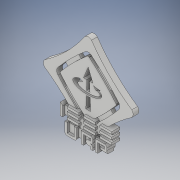
# Autodesk Inventor part: IEEE 3D
Saved by Autodesk Inventor 2018 (Build 220112000, 112)
## iProperties
Created: 2017-04-26
Part Number: IEEE 3D
Material: Generic
Document SubType Name: Modeling
Designer: Docente
Density: 1 g/cm^3
Appearance: Default
Author: Docente
Autodesk Inventor part; units mm, degrees
ref_plane "XY Plane" through (0, 0, 0) normal (0, 0, 1) x (1, 0, 0)
sketch "Sketch1" plane through (0, 0, 0) normal (0, 0, 1) x (1, 0, 0)
  line L0 (0, 0) -> (40, 0) construction
  line L1 (40, 0) -> (40, 40) construction
  line L2 (40, 40) -> (0, 40) construction
  line L3 (0, 40) -> (0, 0) construction
  line L4 (21.4142, 38.5858) -> (38.5858, 21.4142)
  line L5 (21.4142, 1.4142) -> (38.5858, 18.5858)
  line L6 (18.5858, 1.4142) -> (1.4142, 18.5858)
  line L7 (18.5858, 38.5858) -> (1.4142, 21.4142)
  arc A0 (21.4142, 38.5858) -> (18.5858, 38.5858) centre (20, 37.1716) ccw
  arc A1 (38.5858, 18.5858) -> (38.5858, 21.4142) centre (37.1716, 20) ccw
  arc A2 (18.5858, 1.4142) -> (21.4142, 1.4142) centre (20, 2.8284) ccw
  arc A3 (1.4142, 21.4142) -> (1.4142, 18.5858) centre (2.8284, 20) ccw
  line L8 (20, 0) -> (20, 20) construction
  line L9 (20, 20) -> (40, 20) construction
  line L10 (20, 20) -> (76.5685, 76.5685) construction
  line L11 (20, 20) -> (100, 20) construction
  line L12 (20, 20) -> (76.5685, -36.5685) construction
  line L13 (20, 20) -> (100, 20) construction
  line L14 (20, 20) -> (-36.5685, 76.5685) construction
  line L15 (20, 20) -> (100, 20) construction
  line L16 (20, 20) -> (-36.5685, -36.5685) construction
  line L17 (20, 20) -> (100, 20) construction
  line L18 (37.1716, 20) -> (38.5858, 21.4142) construction
  line L19 (37.1716, 20) -> (38.5858, 18.5858) construction
  line L20 (20, 37.1716) -> (21.4142, 38.5858) construction
  line L21 (20, 37.1716) -> (18.5858, 38.5858) construction
  circle A4 centre (76.5685, 76.5685) radius 66.9678
  circle A5 centre (76.5685, -36.5685) radius 66.9678
  circle A6 centre (-36.5685, -36.5685) radius 66.9678
  circle A7 centre (-36.5685, 76.5685) radius 66.9678
  point P0 (20, 40)
  point P1 (20, 0)
  point P2 (0, 20)
  dimension "d0" = 40
  dimension "d1" = 40
  dimension "d7" = 2
  dimension "d8" = 20
  dimension "d13" = 20
  dimension "d14" = 80
  dimension "d15" = 45
  dimension "d16" = 80
  dimension "d17" = 45
  dimension "d18" = 80
  dimension "d19" = 135
  dimension "d20" = 80
  dimension "d21" = 135
  constraints: 44 end point, 8 point on circle, 8 point on line, 8 tangent, 5 horizontal, 4 centre point, 4 coincident, 4 equal length, 4 midpoint, 3 equal radius, 2 parallel, 2 perpendicular, 1 vertical, 12 other
  measures "d0" distance of L2.end L1.end
  measures "d1" distance of L1.end L0.end
  measures "d7" radius of A0
  measures "d8" distance between parallel lines of L3 L8
  measures "d13" distance between parallel lines of L0 L9
  measures "d14" distance of L8.end L10.end
  measures "d15" angle of L11 L10
  measures "d16" distance of L8.end L12.end
  measures "d17" angle of L12 L13
  measures "d18" distance of L8.end L14.end
  measures "d19" angle of L15 L14
  measures "d20" distance of L8.end L16.end
  measures "d21" angle of L16 L17
extrude "Extrusion3" add sketch "Sketch1" along normal blind 2.5 contours A4 A1 A5 A2 A6 A3 A7 A0 | L4 A4 | A7 L7 | L5 A5 | A6 L6
extrude "Extrusion4" cut sketch "Sketch1" along normal blind 3.5 contours A4 A7 A5 L4 | L4 A4 | A7 L7 | L7 A7 A6 A4 | A4 A7 | A5 A4 A6 L5 | L5 A5 | A5 A4 | A6 L6 | L6 A6 A5 A7 | A7 A6 | A6 A5
ref_plane "Work Plane1" through (20, 0, 0) normal (1, 0, 0) x (0, 1, 0)
sketch "Sketch6" plane through (0, 0, 2.5) normal (0, 0, 1) x (1, 0, 0)
  line L0 (18.5858, 38.5858) -> (1.4142, 21.4142) construction
  line L1 (18.5858, 1.4142) -> (1.4142, 18.5858) construction
  line L2 (21.4142, 1.4142) -> (38.5858, 18.5858) construction
  line L3 (21.4142, 38.5858) -> (38.5858, 21.4142) construction
  arc A0 (21.4142, 38.5858) -> (18.5858, 38.5858) centre (20, 37.1716) ccw construction
  arc A1 (1.4142, 21.4142) -> (1.4142, 18.5858) centre (2.8284, 20) ccw construction
  arc A2 (18.5858, 1.4142) -> (21.4142, 1.4142) centre (20, 2.8284) ccw construction
  arc A3 (38.5858, 18.5858) -> (38.5858, 21.4142) centre (37.1716, 20) ccw construction
  line L4 (2.8284, 20) -> (20, 37.1716) construction
  line L5 (20, 37.1716) -> (37.1716, 20) construction
  line L6 (20, 2.8284) -> (37.1716, 20) construction
  line L7 (20, 2.8284) -> (2.8284, 20) construction
  line L8 (18.5858, 32.9289) -> (7.0711, 21.4142) construction
  line L9 (7.0711, 18.5858) -> (18.5858, 7.0711) construction
  line L10 (21.4142, 7.0711) -> (32.9289, 18.5858) construction
  line L11 (32.9289, 21.4142) -> (21.4142, 32.9289) construction
  arc A4 (21.4142, 32.9289) -> (18.8688, 33.1641) centre (20, 31.5147) ccw
  arc A5 (33.1641, 18.8688) -> (33.1641, 21.1312) centre (31.5147, 20) ccw
  arc A6 (18.8688, 6.8359) -> (21.4142, 7.0711) centre (20, 8.4853) ccw
  arc A7 (7.0711, 21.4142) -> (7.0711, 18.5858) centre (8.4853, 20) ccw
  line L12 (20, 31.5147) -> (20, 8.4853) construction
  line L13 (8.4853, 20) -> (31.5147, 20) construction
  line L14 (20, 20) -> (76.5685, 76.5685) construction
  line L15 (20, 20) -> (100, 20) construction
  arc A8 (7.0711, 18.5858) -> (18.8688, 6.8359) centre (76.5685, 76.5685) ccw
  line L16 (20, 20) -> (-36.5685, 76.5685) construction
  arc A9 (21.4142, 7.0711) -> (33.1641, 18.8688) centre (-36.5685, 76.5685) ccw
  line L17 (20, 20) -> (-36.5685, -36.5685) construction
  line L18 (20, 20) -> (76.5685, -36.5685) construction
  arc A10 (18.8688, 33.1641) -> (7.0711, 21.4142) centre (76.5685, -36.5685) ccw
  arc A11 (33.1641, 21.1312) -> (21.4142, 32.9289) centre (-36.5685, -36.5685) ccw
  point P0 (0, 0)
  dimension "d41" = 2
  dimension "d42" = 2
  dimension "d43" = 80
  dimension "d44" = 45
  constraints: 30 end point, 16 point on circle, 8 centre point, 8 tangent, 6 perpendicular, 4 coincident, 3 equal radius, 3 symmetric about line, 2 horizontal, 1 equal length, 1 midpoint, 1 vertical, 3 other
  measures "d41" distance between parallel lines of L4 L8
  measures "d42" radius of A4
  measures "d43" distance of L14.start L14.end
  measures "d44" angle of L15 L14
sketch "Sketch7" plane through (20, 0, 0) normal (1, 0, 0) x (0, 1, 0)
  line L0 (33.5147, 2.5) -> (32.9289, 2.5) construction
  line L1 (33.5147, 2.5) -> (32.0147, 2.5)
  line L2 (32.0147, 2.5) -> (32.0147, -1)
  line L3 (32.0147, -1) -> (33.5147, -1)
  line L4 (33.5147, -1) -> (33.5147, 2.5)
  point P0 (0, 0)
  point P1 (33.1641, 2.5)
  dimension "d45" = 1.5
  dimension "d46" = 3.5
  constraints: 8 end point, 2 parallel, 1 horizontal, 1 perpendicular
  measures "d45" distance of L3.end L2.end
  measures "d46" distance of L2.end L1.end
sweep "Sweep1" cut profiles "Sketch7" path "Sketch6" path curves A4 A11 A5 A9 A6 A8 A7 A10
sketch "Sketch8" plane through (0, 0, 2.5) normal (0, 0, 1) x (1, 0, 0)
  line L0 (20, 20) -> (-36.5685, 76.5685) construction
  line L1 (20, 20) -> (76.5685, -36.5685) construction
  line L2 (20, 20) -> (-36.5685, -36.5685) construction
  line L3 (20, 20) -> (76.5685, 76.5685) construction
  line L4 (20, 20) -> (11.3989, 28.6011)
  line L5 (20, 31.5147) -> (20, 8.4853) construction
  line L6 (20, 20) -> (76.5685, 76.5685) construction
  point P0 (0, 0)
  constraints: 4 end point, 1 point on line
ref_plane "Work Plane2" through (11.3989, 28.6011, 2.5) normal (-0.7071068, 0.7071068, 0) x (-0.7071068, -0.7071068, 0)
sketch "Sketch9" plane through (11.3989, 28.6011, 2.5) normal (-0.7071068, 0.7071068, 0) x (-0.7071068, -0.7071068, 0)
  line L0 (0, -0.5) -> (0, 0)
  line L1 (-4, -2) -> (4, -2)
  line L2 (4, -2) -> (4, -0.5)
  line L3 (4, -0.5) -> (-4, -0.5)
  line L4 (-4, -0.5) -> (-4, -2)
  point P0 (28.2843, -2.5)
  dimension "d52" = 0.5
  dimension "d53" = 8
  dimension "d54" = 1.5
  constraints: 10 end point, 2 parallel, 1 coincident, 1 horizontal, 1 midpoint, 1 perpendicular, 1 vertical
  measures "d52" distance of L0.start L0.end
  measures "d53" distance of L3.end L2.end
  measures "d54" distance of L2.end L1.end
sweep "Sweep2" add profiles "Sketch9" path "Sketch8"
mirror "Mirror1" about plane through (20, 0, 0) normal (1, 0, 0) of "Sweep2"
ref_plane "Work Plane3" through (0, 20, 0) normal (0, 1, 0) x (-1, 0, 0)
mirror "Mirror2" about plane through (0, 20, 0) normal (0, 1, 0) of "Sweep2", "Mirror1"
sketch "Sketch10" plane through (20, 0, 0) normal (1, 0, 0) x (0, 1, 0)
  point P0 (0, 0)
sketch "Sketch11" plane through (0, 0, 2.5) normal (0, 0, 1) x (1, 0, 0)
  line L0 (20, 28) -> (20, 12) construction
  line L1 (19, 12) -> (21, 12)
  line L2 (19.5, 25) -> (20.5, 25) construction
  line L3 (20, 28) -> (20, 25) construction
  line L4 (21, 12) -> (20.5, 25)
  line L5 (19, 12) -> (19.5, 25)
  line L6 (20, 28) -> (25.5169, 28) construction
  line L7 (20, 28) -> (20, 23) construction
  line L8 (20, 23) -> (18, 23)
  line L9 (18, 23) -> (20, 28)
  line L10 (20, 23) -> (22, 23)
  line L11 (22, 23) -> (20, 28)
  line L12 (19.4231, 23) -> (20.5769, 23)
  line L13 (20, 20) -> (20, 18.7353) construction
  arc A0 (19.2704, 19.0296) -> (20.7296, 19.0296) centre (20, 28) ccw
  arc A1 (19.1934, 17.0296) -> (20.8066, 17.0296) centre (20, 28) ccw
  line L14 (19.2704, 19.0296) -> (19.4231, 23)
  line L15 (19.4231, 23) -> (20.5769, 23)
  line L16 (20.5769, 23) -> (20.7296, 19.0296)
  line L17 (19, 12) -> (19.1934, 17.0296)
  line L18 (20.8066, 17.0296) -> (21, 12)
  line L19 (19, 12) -> (21, 12)
  line L20 (21, 12) -> (20.8066, 17.0296)
  point P0 (0, 0)
  dimension "d58" = 16
  dimension "d59" = 2
  dimension "d60" = 1
  dimension "d61" = 3
  dimension "d65" = 5
  dimension "d66" = 2
  dimension "d88" = 9
  dimension "d89" = 11
  constraints: 42 end point, 9 point on line, 7 collinear, 4 horizontal, 4 point on circle, 3 coincident, 3 midpoint, 2 centre point, 1 symmetric about line, 1 vertical
  measures "d58" distance of L0.end L0.start
  measures "d59" distance of L1.start L1.end
  measures "d60" distance of L2.start L2.end
  measures "d61" distance of L3.end L0.start
  measures "d65" distance of L0.start L7.end
  measures "d66" distance of L7.end L8.end
  measures "d88" radius of A0
  measures "d89" radius of A1
sketch "Sketch12" plane through (0, 0, 2.5) normal (0, 0, 1) x (1, 0, 0)
  line L0 (21, 12) -> (20.5, 25) construction
  ellipse E0 centre (20.3, 20) end of major axis (25.0589, 20) minor radius 1.6476 (17.6355, 21.3651) -> (21.5863, 21.5863) ccw
  ellipse E1 centre (19.6, 20) end of major axis (13.4024, 20) minor radius 2.3878 (16.4416, 22.0545) -> (22.1724, 22.1724) ccw
  line L1 (20, 20) -> (20.3, 20) construction
  line L2 (20, 20) -> (19.6, 20) construction
  line L3 (20, 20) -> (16.4718, 22.037) construction
  line L4 (20, 20) -> (24.074, 20) construction
  line L5 (17.6355, 21.3651) -> (16.4416, 22.0545) construction
  line L6 (22.1724, 22.1724) -> (25.1343, 21.6955)
  line L7 (19.9483, 19.9104) -> (22.2046, 22.1667) construction
  line L8 (19.9483, 19.9104) -> (23.1392, 19.9104) construction
  line L9 (20, 20) -> (22.465, 22.465) construction
  line L10 (20, 20) -> (23.486, 20) construction
  line L11 (22.1724, 22.1724) -> (23.4452, 20.8996)
  line L12 (22.1724, 22.1724) -> (23.9724, 22.1724) construction
  line L13 (23.4452, 20.8996) -> (25.1343, 21.6955)
  line L14 (16.4416, 22.0545) -> (17.6355, 21.3651)
  line L15 (23.858, 21.0941) -> (24.5669, 21.4281)
  point P0 (0, 0)
  dimension "d72" = 6.1976
  dimension "d73" = 2.3878
  dimension "d74" = 4.7589
  dimension "d75" = 1.6476
  dimension "d70" = 0.3
  dimension "d71" = 0.4
  dimension "d76" = 150
  dimension "d77" = 3
  dimension "d78" = 45
  dimension "d79" = 45
  dimension "d80" = 2.9619
  dimension "d81" = 1.8
  dimension "d82" = 45
  constraints: 30 end point, 6 horizontal, 6 point on line, 4 equal length, 2 coincident, 1 collinear, 11 other
  measures "d70" distance of L1.start L1.end
  measures "d71" distance of L1.start L2.end
  measures "d76" angle of L4 L3
  measures "d77" distance of L6.start L6.end
  measures "d78" angle of L8 L7
  measures "d79" angle of L10 L9
  measures "d80" horizontal distance of L6.start L6.end
  measures "d81" distance of L6.start L11.end
  measures "d82" angle of L11 L12
extrude "Extrusion7" cut sketch "Sketch11" against normal blind 4 contours L5 A1 L4 L1 | L5 L8 L10 L4 A0 | L8 L9 L11 L10
extrude "Extrusion8" cut sketch "Sketch12" against normal blind 4
sketch "Sketch14" plane through (0, 0, 2.5) normal (0, 0, 1) x (1, 0, 0)
  line L0 (9, 20) -> (31, 20) construction
  line L1 (31, 20) -> (31, 5) construction
  line L2 (31, 5) -> (9, 5) construction
  line L3 (9, 5) -> (9, 20) construction
  line L4 (9, 5) -> (10, 5)
  line L5 (10, 5) -> (10, 9)
  line L6 (9, 10) -> (9, 10)
  line L7 (9, 10) -> (9, 5)
  arc A0 (10, 9) -> (9, 10) centre (9, 9) ccw
  line L8 (12, 6) -> (17, 6)
  line L9 (17, 6) -> (17, 5)
  line L10 (17, 5) -> (12, 5)
  line L11 (12, 5) -> (12, 6)
  line L12 (12, 8) -> (17, 8)
  line L13 (17, 8) -> (17, 7)
  line L14 (17, 7) -> (12, 7)
  line L15 (12, 7) -> (12, 8)
  line L16 (12, 10) -> (17, 10)
  line L17 (17, 10) -> (17, 9)
  line L18 (17, 9) -> (12, 9)
  line L19 (12, 9) -> (12, 10)
  line L20 (38.5, 5) -> (3.5, 5) construction
  line L21 (17, 5) -> (17, 6)
  line L22 (17, 5) -> (18, 5) construction
  line L23 (18, 5) -> (18, 9.9034) construction
  line L24 (18, 5) -> (22.9034, 5) construction
  line L25 (24, 6) -> (19, 6)
  line L26 (19, 6) -> (19, 5)
  line L27 (19, 5) -> (24, 5)
  line L28 (24, 5) -> (24, 6)
  line L29 (24, 7) -> (24, 8)
  line L30 (24, 8) -> (19, 8)
  line L31 (19, 8) -> (19, 7)
  line L32 (19, 7) -> (24, 7)
  line L33 (24, 9) -> (24, 10)
  line L34 (24, 10) -> (19, 10)
  line L35 (19, 10) -> (19, 9)
  line L36 (19, 9) -> (24, 9)
  line L37 (19, 5) -> (19, 6)
  line L38 (24, 5) -> (25, 5) construction
  line L39 (25, 5) -> (25, 9.5) construction
  line L40 (26, 9) -> (26, 10)
  line L41 (31, 7) -> (26, 7)
  line L42 (26, 8) -> (31, 8)
  line L43 (31, 9) -> (26, 9)
  line L44 (26, 10) -> (31, 10)
  line L45 (31, 5) -> (26, 5)
  line L46 (26, 6) -> (31, 6)
  line L47 (31, 8) -> (31, 7)
  line L48 (31, 6) -> (31, 5)
  line L49 (31, 5) -> (31, 6)
  line L50 (31, 10) -> (31, 9)
  line L51 (26, 7) -> (26, 8)
  line L52 (26, 5) -> (26, 6)
  line L53 (9, 20) -> (31, 20) construction
  line L54 (31, 20) -> (31, -1) construction
  line L55 (15, -1) -> (12, -1) construction
  line L56 (9, -1) -> (9, 20) construction
  line L57 (11, 4) -> (12, 4)
  line L58 (12, 4) -> (12, 0)
  line L59 (12, -1) -> (11, -1) construction
  line L60 (11, 0) -> (11, 4)
  line L61 (11, 0) -> (16, 0)
  line L62 (16, 0) -> (16, 0)
  line L63 (16, -1) -> (11, -1) construction
  line L64 (11, -1) -> (11, 0)
  line L65 (16, -1) -> (16, 0)
  line L66 (16, -1) -> (15, -1) construction
  line L67 (15, 0) -> (15, 4) construction
  line L68 (15, 4) -> (16, 4) construction
  line L69 (16, 4) -> (16, -1) construction
  line L70 (18, 4) -> (19, 4)
  line L71 (19, 4) -> (19, -1)
  line L72 (19, -1) -> (18, -1)
  line L73 (18, -1) -> (18, 4)
  line L74 (18, 4) -> (22, 4)
  line L75 (23, 3) -> (23, 3)
  line L76 (23, 3) -> (18, 3)
  line L77 (18, 3) -> (18, 4)
  line L78 (23, 3) -> (23, 4)
  line L79 (22, 3) -> (23, 3)
  line L80 (23, 3) -> (23, 2)
  line L81 (22, 1) -> (22, 1)
  line L82 (22, 1) -> (22, 3)
  arc A1 (23, 3) -> (22, 4) centre (22, 3) ccw
  arc A2 (22, 1) -> (23, 2) centre (22, 2) ccw
  line L83 (22, 2) -> (21, 2)
  line L84 (20, 1) -> (20, 1)
  line L85 (21, 0) -> (22, 0)
  line L86 (22, 0) -> (22, 2)
  arc A3 (21, 2) -> (20, 1) centre (21, 1) ccw
  arc A4 (20, 1) -> (21, 0) centre (21, 1) ccw
  line L87 (22, 1) -> (22, 1)
  line L88 (23, 0) -> (23, -1)
  line L89 (23, -1) -> (22, -1)
  line L90 (22, -1) -> (22, 1)
  arc A5 (23, 0) -> (22, 1) centre (22, 0) ccw
  arc A6 (15, -1) -> (16, 0) centre (15, 0) ccw
  arc A7 (11, 0) -> (12, -1) centre (12, 0) ccw
  line L91 (25, 4) -> (24, 4)
  line L92 (24, 4) -> (24, -1)
  line L93 (24, -1) -> (25, -1)
  line L94 (25, -1) -> (25, 4)
  line L95 (24, 4) -> (28, 4)
  line L96 (29, 3) -> (29, 3)
  line L97 (29, 3) -> (24, 3)
  line L98 (24, 3) -> (24, 4)
  arc A8 (29, 3) -> (28, 4) centre (28, 3) ccw
  line L99 (28, 3) -> (29, 3)
  line L100 (29, 3) -> (29, 2)
  line L101 (28, 1) -> (28, 1)
  line L102 (28, 1) -> (28, 3)
  arc A9 (28, 1) -> (29, 2) centre (28, 2) ccw
  line L103 (28, 2) -> (26, 2)
  line L104 (26, 2) -> (26, 2)
  line L105 (27, 1) -> (28, 1)
  line L106 (28, 1) -> (28, 2)
  arc A10 (26, 2) -> (27, 1) centre (27, 2) ccw
  line L107 (15, -1) -> (12, -1)
  line L108 (15, 4) -> (16, 4)
  line L109 (16, 4) -> (16, 0)
  line L110 (16, 0) -> (15, 0)
  line L111 (15, 0) -> (15, 4)
  point P0 (0, 0)
  point P1 (20, 20)
  point P2 (9, 5)
  point P3 (20, 20)
  point P4 (23, 4)
  point P5 (20, 2)
  point P6 (23, 1)
  dimension "d96" = 22
  dimension "d97" = 15
  dimension "d98" = 5
  dimension "d99" = 1
  dimension "d100" = 0
  dimension "d101" = 1
  dimension "d102" = 5
  dimension "d103" = 1
  dimension "d104" = 2
  dimension "d105" = 5
  dimension "d106" = 1
  dimension "d109" = 1
  dimension "d110" = 5
  dimension "d111" = 1
  dimension "d114" = 1
  dimension "d129" = 1
  dimension "d130" = 1
  dimension "d131" = 90
  dimension "d132" = 1
  dimension "d136" = 22
  dimension "d137" = 21
  dimension "d138" = 5
  dimension "d139" = 1
  dimension "d140" = 2
  dimension "d141" = 5
  dimension "d142" = 1
  dimension "d143" = 1
  dimension "d146" = 1
  dimension "d147" = 1
  dimension "d148" = 2
  dimension "d149" = 5
  dimension "d150" = 1
  dimension "d151" = 1
  dimension "d154" = 1
  dimension "d155" = 2
  dimension "d156" = 1
  dimension "d157" = 1
  dimension "d158" = 2
  dimension "d159" = 2
  dimension "d160" = 1
  dimension "d161" = 2
  dimension "d162" = 1
  dimension "d163" = 1
  dimension "d164" = 2
  dimension "d165" = 1
  dimension "d166" = 5
  dimension "d167" = 1
  dimension "d171" = 2
  dimension "d172" = 1
  dimension "d173" = 1
  dimension "d174" = 2
  dimension "d175" = 1
  dimension "d176" = 1
  constraints: 224 end point, 38 parallel, 26 symmetric about line, 24 tangent, 23 collinear, 22 point on circle, 21 perpendicular, 20 horizontal, 16 point on line, 11 centre point, 3 vertical, 2 equal radius, 2 midpoint, 1 coincident
  measures "d96" distance of L1.end L2.end
  measures "d97" distance of L0.end L1.end
  measures "d98" distance of L6.end L4.start
  measures "d99" distance between parallel lines of L5 L7
  measures "d100" distance between parallel lines of L3 L7
  measures "d101" radius of A0
  measures "d102" distance of L8.start L8.end
  measures "d103" distance between parallel lines of L8 L10
  measures "d104" distance between parallel lines of L5 L11
  measures "d105" distance of L15.end L12.end
  measures "d106" distance between parallel lines of L12 L14
  measures "d109" distance between parallel lines of L8 L14
  measures "d110" distance of L19.end L16.end
  measures "d111" distance between parallel lines of L16 L18
  measures "d114" distance between parallel lines of L12 L18
  measures "d129" distance of L9.end L21.end
  measures "d130" distance of L9.end L22.end
  measures "d131" angle of L24 L23
  measures "d132" distance of L27.end L38.end
  measures "d136" distance of L54.end L56.start
  measures "d137" distance between parallel lines of L0 L55
  measures "d138" distance of L59.end L57.start
  measures "d139" distance between parallel lines of L60 L58
  measures "d140" distance between parallel lines of L56 L60
  measures "d141" distance of L61.start L62.start
  measures "d142" distance between parallel lines of L61 L63
  measures "d143" distance of L63.start L65.end
  measures "d146" distance between parallel lines of L69 L67
  measures "d147" distance between parallel lines of L73 L71
  measures "d148" distance between parallel lines of L69 L73
  measures "d149" distance of L74.start point (23, 4)
  measures "d150" distance between parallel lines of L74 L76
  measures "d151" distance of L75.end L78.end
  measures "d154" radius of A1
  measures "d155" distance of L81.end L79.start
  measures "d156" distance between parallel lines of L80 L82
  measures "d157" radius of A2
  measures "d158" distance between parallel lines of L85 L83
  measures "d159" distance of L83.start point (20, 2)
  measures "d160" radius of A3
  measures "d161" distance of point (23, 1) L88.end
  measures "d162" radius of A5
  measures "d163" radius of A6
  measures "d164" distance between parallel lines of L80 L94
  measures "d165" distance between parallel lines of L94 L92
  measures "d166" distance of L96.end L97.end
  measures "d167" radius of A8
  measures "d171" distance of L101.end L99.start
  measures "d172" distance between parallel lines of L102 L100
  measures "d173" radius of A9
  measures "d174" distance of L103.start L103.end
  measures "d175" distance between parallel lines of L105 L103
  measures "d176" radius of A10
extrude "Extrusion10" add sketch "Sketch14" along normal blind 1 and the other way blind 2.5
sketch "Sketch15" plane through (0, 0, 2.5) normal (0, 0, 1) x (1, 0, 0)
  line L0 (7.5, 20) -> (32.5, 20) construction
  line L1 (32.5, 20) -> (32.5, -15) construction
  line L2 (32.5, -15) -> (7.5, -15) construction
  line L3 (7.5, -15) -> (7.5, 20) construction
  line L4 (9.5, 9) -> (16.5, 9)
  line L5 (16.5, 9) -> (16.5, 5.5)
  line L6 (16.5, 5.5) -> (9.5, 5.5)
  line L7 (9.5, 5.5) -> (9.5, 9)
  line L8 (20, 41.9997) -> (20, -1.9997) construction
  line L9 (20, 41.9997) -> (63.9994, 41.9997) construction
  line L10 (30.5, 9) -> (23.5, 9)
  line L11 (23.5, 9) -> (23.5, 5.5)
  line L12 (23.5, 5.5) -> (30.5, 5.5)
  line L13 (30.5, 5.5) -> (30.5, 9)
  line L14 (11.6, 3.5) -> (28.4, 3.5)
  line L15 (28.4, 3.5) -> (28.4, 0)
  line L16 (28.4, 0) -> (11.6, 0)
  line L17 (11.6, 0) -> (11.6, 3.5)
  point P0 (0, 0)
  point P1 (20, 20)
  point P2 (20, 20)
  point P3 (20, 3.5)
  dimension "d181" = 35
  dimension "d182" = 25
  dimension "d183" = 7
  dimension "d184" = 3.5
  dimension "d185" = 2
  dimension "d186" = 11
  dimension "d187" = 90
  dimension "d188" = 3.5
  dimension "d189" = 16.8
  dimension "d190" = 5.5
  constraints: 36 end point, 6 parallel, 4 horizontal, 4 perpendicular, 4 symmetric about line, 3 midpoint, 1 coincident, 1 point on line
  measures "d181" distance of L0.end L1.end
  measures "d182" distance of L1.end L2.end
  measures "d183" distance of L4.start L4.end
  measures "d184" distance of L4.end L5.end
  measures "d185" distance between parallel lines of L3 L7
  measures "d186" distance between parallel lines of L0 L4
  measures "d187" angle of L8 L9
  measures "d188" distance of L16.end L14.start
  measures "d189" distance of L15.end L16.end
  measures "d190" distance between parallel lines of L14 L4
extrude "Extrusion11" add sketch "Sketch15" against normal blind 2.5
equation "\"d99\" = 0.2 * d98"
equation "\"d101\" = d99"
equation "\"d102\" = d98"
equation "\"d103\" = d99"
equation "\"d104\" = 2 * d99"
equation "\"d109\" = d99"
equation "\"d114\" = d99"
equation "\"d129\" = d99"
equation "\"d130\" = d99"
equation "\"d132\" = d99"
equation "\"d108\" = 0.2 * d107"
equation "\"d113\" = 0.2 * d112"
equation "\"d107\" = 3"
equation "\"d112\" = 3"
body "Solid3"
